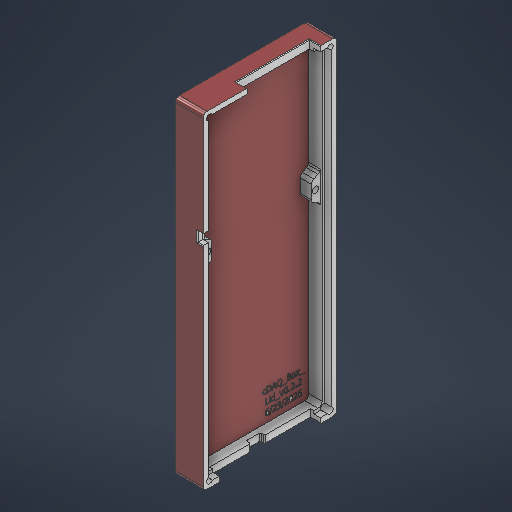
# Autodesk Inventor part: cDAQ_Box_Lid_v0.2.2ipt
Saved by Autodesk Inventor 2027 (Build 310192000, 192)
## iProperties
Created: 2026-05-08
Part Number: cDAQ_Box_Lid_v0.2.2ipt
Material: Generic
Document SubType Name: Modeling
Designer: giese
Density: 1 g/cm^3
Appearance: Default
Author: giese
Autodesk Inventor part; units mm, degrees
(part 1 of 2)
ref_plane "YZ Plane" through (0, 0, 0) normal (1, 0, 0) x (0, 1, 0)
ref_plane "XZ Plane" through (0, 0, 0) normal (0, 1, 0) x (-1, 0, 0)
ref_plane "XY Plane" through (0, 0, 0) normal (0, 0, 1) x (1, 0, 0)
sketch "Sketch1" plane through (0, 0, 0) normal (1, 0, 0) x (0, 1, 0)
  line L0 (50.7569, 48.4212) -> (-204.2591, 48.4212)
  line L1 (-204.2591, 48.4212) -> (-204.2591, -55.7188)
  line L2 (-204.2591, -55.7188) -> (50.7569, -55.7188)
  line L3 (50.7569, -55.7188) -> (50.7569, 48.4212)
  point P0 (0, 0)
  dimension "d0" = 104.14
  dimension "d1" = 255.016
  constraints: 8 end point, 2 parallel, 1 horizontal, 1 perpendicular
  measures "d0" distance of L2.end L0.start
  measures "d1" distance of L0.start L0.end
extrude "Extrusion1" add sketch "Sketch1" along normal blind 21.59
sketch "Sketch2" plane through (21.59, 0, 0) normal (1, 0, 0) x (0, 0, -1)
  line L0 (-42.0712, 44.4069) -> (49.3688, 44.4069)
  line L1 (49.3688, 44.4069) -> (49.3688, -197.9091)
  line L2 (49.3688, -197.9091) -> (-42.0712, -197.9091)
  line L3 (-42.0712, -197.9091) -> (-42.0712, 44.4069)
  line L4 (-48.4212, 50.7569) -> (-48.4212, -204.2591) projected
  line L5 (-48.4212, -204.2591) -> (55.7188, -204.2591) projected
  point P0 (0, 0)
  dimension "d4" = 91.44
  dimension "d5" = 242.316
  dimension "d6" = 6.35
  dimension "d7" = 6.35
  constraints: 8 end point, 2 parallel, 1 horizontal, 1 perpendicular
  measures "d4" distance of L0.start L0.end
  measures "d5" distance of L0.end L1.end
  measures "d6" distance between parallel lines of L4 L3
  measures "d7" distance between parallel lines of L5 L2
extrude "Extrusion2" cut sketch "Sketch2" against normal blind 15.24
sketch "Sketch3" plane through (0, 0, 0) normal (-1, 0, 0) x (0, 0, 1)
  circle A0 centre (-32.8588, 7.3229) radius 2
  line L0 (-55.7188, -204.2591) -> (-55.7188, 50.7569) projected
  line L1 (-55.7188, 50.7569) -> (48.4212, 50.7569) projected
  circle A1 centre (-14.36, 7.3229) radius 2
  circle A2 centre (4.1389, 7.3229) radius 2
  point P0 (0, 0)
  dimension "d10" = 22.86
  dimension "d11" = 43.434
  dimension "d12" = 43.434
  dimension "d13" = 18.4988
  dimension "d14" = 4
  dimension "d15" = 4
  dimension "d16" = 43.434
  dimension "d17" = 18.4988
  dimension "d18" = 36.9976
  dimension "d21" = 4
  constraints: 3 centre point
  measures "d10" distance from line of L0 A0.centre
  measures "d11" distance from line of L1 A0.centre
  measures "d12" distance from line of L1 A1.centre
  measures "d13" distance of A0.centre A1.centre
  measures "d14" diameter of A1
  measures "d15" diameter of A2
  measures "d16" distance from line of L1 A2.centre
  measures "d17" distance of A1.centre A2.centre
  measures "d18" distance of A0.centre A2.centre
  measures "d21" diameter of A0
extrude "Extrusion3" [suppressed]
sketch "Sketch6" plane through (0, 50.7569, 48.4212) normal (0, 1, 0) x (1, 0, 0)
  line L0 (21.59, 6.35) -> (21.59, 97.79) projected
  line L1 (12.954, 34.29) -> (21.59, 34.29)
  line L2 (21.59, 34.29) -> (21.59, 91.44)
  line L3 (21.59, 91.44) -> (12.954, 91.44)
  line L4 (12.954, 91.44) -> (12.954, 34.29)
  line L5 (0, 104.14) -> (21.59, 104.14) projected
  point P0 (0, 48.4212)
  point P1 (17.272, 91.44)
  point P2 (17.272, 34.29)
  dimension "d30" = 8.636
  dimension "d32" = 12.7
  dimension "d220" = 69.85
  constraints: 8 end point, 2 midpoint, 2 parallel, 1 horizontal, 1 perpendicular, 1 point on line
  measures "d30" distance between parallel lines of L0 L4
  measures "d32" distance between parallel lines of L5 L3
  measures "d220" distance between parallel lines of L5 L1
extrude "Extrusion5" cut sketch "Sketch6" against normal blind 6.35
fillet "Fillet1" radius 3.175 4 edges at (10.795, 50.7569, -55.7188) (10.795, 50.7569, 48.4212) (10.795, -204.2591, 48.4212) (10.795, -204.2591, -55.7188)
sketch "Sketch7" plane through (21.59, 0, 0) normal (1, 0, 0) x (0, 0, -1)
  line L0 (-42.0712, -197.9091) -> (-42.0712, 44.4069) projected
  line L1 (-42.0712, 44.4069) -> (-42.3252, 44.4069)
  line L2 (-42.3252, 46.6929) -> (-44.2302, 46.6929)
  line L3 (-44.2302, 46.6929) -> (-44.2302, 51.0109)
  line L4 (-42.0712, -190.1621) -> (-42.0712, -197.9091)
  line L5 (49.3688, -197.9091) -> (-42.0712, -197.9091) projected
  line L6 (-40.4202, -200.1951) -> (-44.2302, -200.1951)
  line L7 (-44.2302, -200.1951) -> (-44.2302, -190.1621)
  line L8 (49.3688, 44.4069) -> (49.3688, -197.9091) projected
  line L9 (49.3688, -192.7021) -> (49.3688, -197.9091)
  line L10 (49.3688, -197.9091) -> (43.9078, -197.9091)
  line L11 (49.3688, -197.9091) -> (49.3688, -192.7021)
  line L12 (51.5278, -192.7021) -> (51.5278, -200.1951)
  line L13 (51.5278, -200.1951) -> (43.9078, -200.1951)
  line L14 (-42.0712, 44.4069) -> (49.3688, 44.4069) projected
  line L15 (42.0028, 44.4069) -> (49.3688, 44.4069)
  line L16 (51.5278, 48.4709) -> (51.5278, 46.6929)
  line L17 (51.5278, 46.6929) -> (42.0028, 46.6929)
  line L18 (-42.3252, 46.6929) -> (42.0028, 46.6929)
  line L19 (42.0028, 44.4069) -> (-42.3252, 44.4069)
  line L20 (51.5278, 48.4709) -> (51.5278, -192.7021)
  line L21 (44.2888, -195.2421) -> (44.2888, 44.4069)
  line L22 (43.9078, -197.9091) -> (-40.4202, -197.9091)
  line L23 (-40.4202, -200.1951) -> (43.9078, -200.1951)
  line L24 (-44.2302, -190.1621) -> (-44.2302, 51.0109)
  line L25 (-42.0712, 44.4069) -> (-42.0712, -190.1621)
  point P0 (0, 0)
  point P1 (-42.0712, 51.0109)
  point P2 (-44.2302, 48.9789)
  point P3 (49.3688, 48.4709)
  point P4 (51.5278, 46.6929)
  point P5 (-44.2302, 46.6929)
  point P6 (-42.0712, 50.7569)
  point P7 (46.8288, 50.7569)
  dimension "d34" = 2.286
  dimension "d35" = 2.159
  dimension "d38" = 2.159
  dimension "d39" = 2.286
  dimension "d42" = 2.286
  dimension "d43" = 2.159
  dimension "d46" = 2.286
  dimension "d47" = 2.159
  constraints: 44 end point, 7 point on line, 4 parallel, 4 perpendicular, 2 collinear, 2 horizontal, 2 vertical, 3 other
  measures "d34" distance between parallel lines of L2 L1
  measures "d35" distance between parallel lines of L0 L3
  measures "d38" distance between parallel lines of L7 L0
  measures "d39" distance between parallel lines of L5 L6
  measures "d42" distance between parallel lines of L5 L13
  measures "d46" distance between parallel lines of L14 L17
extrude "Extrusion6" cut sketch "Sketch7" against normal blind 5 contours L0 L14 L8 L5 | L18 L17 L20 L12 L13 L23 L6 L7 L24 L2
fillet "Fillet2" radius 3.175 6 edges at (11.47, 44.4069, 42.0712) (11.47, 44.4069, -49.3688) (11.47, -197.9091, 42.0712) (19.09, -200.1951, 44.2302) (11.47, -197.9091, -49.3688) (19.09, -200.1951, -51.5278)
sketch "Sketch11" plane through (16.59, 0, 0) normal (1, 0, 0) x (0, 0, -1)
  circle A0 centre (50.6388, 45.6769) radius 2.4005
  line L0 (52.5438, 50.7569) -> (43.0188, 50.7569) projected
  line L1 (55.7188, -201.0841) -> (55.7188, 47.5819) projected
  arc A1 (46.9238, 45.7719) -> (43.7488, 48.9469) centre (43.7488, 45.7719) ccw projected
  circle A2 centre (-43.3412, 45.6769) radius 2.4005
  line L2 (-48.4212, 47.5819) -> (-48.4212, -201.0841) projected
  line L3 (-14.1312, 50.7569) -> (-45.2462, 50.7569) projected
  circle A3 centre (50.6388, -199.1791) radius 2.4005
  line L4 (-45.2462, -204.2591) -> (52.5438, -204.2591) projected
  circle A4 centre (-43.3412, -199.1791) radius 2.4005
  circle A5 centre (45.5588, -50.8431) radius 2.4005
  circle A6 centre (-38.2612, -50.8431) radius 2.4005
  point P0 (0, 0)
  point P1 (45.9939, 48.017)
  point P2 (48.5528, -43.2993)
  point P3 (45.3778, -46.4743)
  point P4 (-30.4007, -42.8803)
  point P5 (-33.5757, -46.0553)
  point P6 (46.8288, 50.7569)
  point P7 (-42.0712, 50.7569)
  dimension "d58" = 4.801
  dimension "d59" = 5.08
  dimension "d60" = 5.08
  dimension "d61" = 4.801
  dimension "d62" = 4.801
  dimension "d63" = 5.08
  dimension "d64" = 5.08
  dimension "d65" = 4.801
  dimension "d66" = 5.08
  dimension "d67" = 5.08
  dimension "d76" = 5.08
  dimension "d77" = 5.08
  dimension "d114" = 4.801
  dimension "d115" = 101.6
  dimension "d116" = 10.16
  dimension "d117" = 4.801
  dimension "d118" = 101.6
  dimension "d119" = 10.16
  constraints: 6 centre point, 1 point on circle
  measures "d58" diameter of A0
  measures "d59" distance from line of L2 A2.centre
  measures "d60" distance from line of L3 A2.centre
  measures "d61" diameter of A2
  measures "d62" diameter of A3
  measures "d63" distance from line of L1 A3.centre
  measures "d64" distance from line of L4 A3.centre
  measures "d65" diameter of A4
  measures "d66" distance from line of L2 A4.centre
  measures "d67" distance from line of L4 A4.centre
  measures "d76" distance from line of L1 A0.centre
  measures "d77" distance from line of L0 A0.centre
  measures "d114" diameter of A5
  measures "d115" distance from line of A5.centre L0
  measures "d116" distance from line of L1 A5.centre
  measures "d117" diameter of A6
  measures "d118" distance from line of A6.centre L3
  measures "d119" distance from line of L2 A6.centre
extrude "Extrusion8" cut sketch "Sketch11" along normal blind 5.08 and the other way blind 17.78
sketch "Sketch13" plane through (6.35, 0, 0) normal (1, 0, 0) x (0, 0, -1)
  line L0 (15.5343, -173.5179) -> (43.4772, -173.5179) construction
  line L1 (43.4772, -173.5179) -> (43.4772, -195.7179) construction
  line L2 (43.4772, -195.7179) -> (15.5343, -195.7179) construction
  line L3 (15.5343, -195.7179) -> (15.5343, -173.5179) construction
  spline S0 degree 2 poles (15.0006, -178.2641) (14.6449, -178.2641) (14.0558, -178.0455) (13.8446, -177.8232) knots 0 0 0 1 2 2 2
  spline S1 degree 2 poles (13.8446, -177.8232) (13.6334, -177.6046) (13.4, -176.9303) (13.4, -176.4783) knots 0 0 0 1 2 2 2
  spline S2 degree 2 poles (13.4, -176.4783) (13.4, -176.0262) (13.6408, -175.3667) (13.8446, -175.1444) knots 0 0 0 1 2 2 2
  spline S3 degree 2 poles (13.8446, -175.1444) (14.0484, -174.9184) (14.6523, -174.6776) (15.0006, -174.6776) knots 0 0 0 1 2 2 2
  spline S4 degree 2 poles (15.0006, -174.6776) (15.2821, -174.6776) (15.8083, -174.8369) (16.012, -174.9407) knots 0 0 0 1 2 2 2
  line L4 (16.012, -174.9407) -> (16.012, -175.5891)
  line L5 (16.012, -175.5891) -> (15.9787, -175.5891)
  spline S5 degree 2 poles (15.9787, -175.5891) (15.9157, -175.5372) (15.723, -175.4038) (15.586, -175.3334) knots 0 0 0 1 2 2 2
  spline S6 degree 2 poles (15.586, -175.3334) (15.4637, -175.2741) (15.1376, -175.1815) (14.9894, -175.1815) knots 0 0 0 1 2 2 2
  spline S7 degree 2 poles (14.9894, -175.1815) (14.5411, -175.1815) (13.9965, -175.8595) (13.9965, -176.4783) knots 0 0 0 1 2 2 2
  spline S8 degree 2 poles (13.9965, -176.4783) (13.9965, -177.0822) (14.5226, -177.7602) (14.9894, -177.7602) knots 0 0 0 1 2 2 2
  spline S9 degree 2 poles (14.9894, -177.7602) (15.271, -177.7602) (15.7823, -177.5268) (15.9787, -177.3452) knots 0 0 0 1 2 2 2
  line L6 (15.9787, -177.3452) -> (16.012, -177.3452)
  line L7 (16.012, -177.3452) -> (16.012, -177.9936)
  spline S10 degree 2 poles (16.012, -177.9936) (15.9268, -178.0344) (15.6675, -178.1492) (15.5637, -178.1752) knots 0 0 0 1 2 2 2
  spline S11 degree 2 poles (15.5637, -178.1752) (15.4155, -178.2196) (15.1821, -178.2641) (15.0006, -178.2641) knots 0 0 0 1 2 2 2
  spline S12 degree 2 poles (20.1876, -175.904) (20.1876, -176.5301) (19.68, -177.5379) (19.2539, -177.8195) knots 0 0 0 1 2 2 2
  spline S13 degree 2 poles (19.2539, -177.8195) (18.9057, -178.0381) (18.1906, -178.1863) (17.6348, -178.1863) knots 0 0 0 1 2 2 2
  line L8 (17.6348, -178.1863) -> (16.5826, -178.1863)
  line L9 (16.5826, -178.1863) -> (16.5826, -173.6143)
  line L10 (16.5826, -173.6143) -> (17.6237, -173.6143)
  spline S14 degree 2 poles (17.6237, -173.6143) (18.2684, -173.6143) (19.002, -173.8069) (19.2613, -173.9774) knots 0 0 0 1 2 2 2
  spline S15 degree 2 poles (19.2613, -173.9774) (19.7022, -174.2701) (20.1876, -175.2371) (20.1876, -175.904) knots 0 0 0 1 2 2 2
  spline S16 degree 2 poles (19.554, -175.8966) (19.554, -175.3705) (19.2058, -174.6257) (18.8612, -174.4146) knots 0 0 0 1 2 2 2
  spline S17 degree 2 poles (18.8612, -174.4146) (18.6167, -174.2701) (18.0646, -174.1404) (17.6534, -174.1404) knots 0 0 0 1 2 2 2
  line L11 (17.6534, -174.1404) -> (17.1902, -174.1404)
  line L12 (17.1902, -174.1404) -> (17.1902, -177.6602)
  line L13 (17.1902, -177.6602) -> (17.6534, -177.6602)
  spline S18 degree 2 poles (17.6534, -177.6602) (18.0572, -177.6602) (18.6685, -177.5305) (18.9168, -177.3563) knots 0 0 0 1 2 2 2
  spline S19 degree 2 poles (18.9168, -177.3563) (19.2354, -177.1415) (19.554, -176.4301) (19.554, -175.8966) knots 0 0 0 1 2 2 2
  line L14 (20.3543, -178.1863) -> (21.8956, -173.6143)
  line L15 (21.8956, -173.6143) -> (22.644, -173.6143)
  line L16 (22.644, -173.6143) -> (24.1853, -178.1863)
  line L17 (24.1853, -178.1863) -> (23.5443, -178.1863)
  line L18 (23.5443, -178.1863) -> (23.1294, -176.908)
  line L19 (23.1294, -176.908) -> (21.3843, -176.908)
  line L20 (21.3843, -176.908) -> (20.9694, -178.1863)
  line L21 (20.9694, -178.1863) -> (20.3543, -178.1863)
  line L22 (22.9627, -176.3893) -> (22.255, -174.2367)
  line L23 (22.255, -174.2367) -> (21.551, -176.3893)
  line L24 (21.551, -176.3893) -> (22.9627, -176.3893)
  spline S20 degree 2 poles (28.4165, -179.3052) (28.2497, -179.3459) (27.8866, -179.3904) (27.7051, -179.3904) knots 0 0 0 1 2 2 2
  spline S21 degree 2 poles (27.7051, -179.3904) (27.1901, -179.3904) (26.5491, -178.8161) (26.5195, -178.2826) knots 0 0 0 1 2 2 2
  spline S22 degree 2 poles (26.5195, -178.2826) (26.4787, -178.2826) (26.4083, -178.2826) (26.3787, -178.2826) knots 0 0 0 1 2 2 2
  spline S23 degree 2 poles (26.3787, -178.2826) (25.9156, -178.2826) (25.1709, -177.9677) (24.9041, -177.6602) knots 0 0 0 1 2 2 2
  spline S24 degree 2 poles (24.9041, -177.6602) (24.641, -177.3563) (24.3595, -176.4671) (24.3595, -175.904) knots 0 0 0 1 2 2 2
  spline S25 degree 2 poles (24.3595, -175.904) (24.3595, -175.326) (24.6447, -174.4516) (24.9078, -174.1404) knots 0 0 0 1 2 2 2
  spline S26 degree 2 poles (24.9078, -174.1404) (25.1746, -173.8329) (25.9193, -173.5179) (26.3787, -173.5179) knots 0 0 0 1 2 2 2
  spline S27 degree 2 poles (26.3787, -173.5179) (26.8455, -173.5179) (27.5939, -173.844) (27.8533, -174.1404) knots 0 0 0 1 2 2 2
  spline S28 degree 2 poles (27.8533, -174.1404) (28.1126, -174.4405) (28.4016, -175.3334) (28.4016, -175.904) knots 0 0 0 1 2 2 2
  spline S29 degree 2 poles (28.4016, -175.904) (28.4016, -176.7932) (27.7088, -177.9492) (27.1049, -178.1529) knots 0 0 0 1 2 2 2
  spline S30 degree 2 poles (27.1049, -178.1529) (27.1197, -178.3234) (27.2086, -178.5975) (27.279, -178.6753) knots 0 0 0 1 2 2 2
  spline S31 degree 2 poles (27.279, -178.6753) (27.3642, -178.7717) (27.5976, -178.8606) (27.8051, -178.8606) knots 0 0 0 1 2 2 2
  spline S32 degree 2 poles (27.8051, -178.8606) (27.9274, -178.8606) (28.2608, -178.7828) (28.3349, -178.7531) knots 0 0 0 1 2 2 2
  line L25 (28.3349, -178.7531) -> (28.4165, -178.7531)
  line L26 (28.4165, -178.7531) -> (28.4165, -179.3052)
  spline S33 degree 2 poles (27.7681, -175.904) (27.7681, -175.4483) (27.5717, -174.748) (27.3939, -174.5183) knots 0 0 0 1 2 2 2
  spline S34 degree 2 poles (27.3939, -174.5183) (27.2123, -174.2812) (26.701, -174.0441) (26.3824, -174.0441) knots 0 0 0 1 2 2 2
  spline S35 degree 2 poles (26.3824, -174.0441) (26.0527, -174.0441) (25.5562, -174.2738) (25.3672, -174.5183) knots 0 0 0 1 2 2 2
  spline S36 degree 2 poles (25.3672, -174.5183) (25.1857, -174.7517) (24.993, -175.4594) (24.993, -175.904) knots 0 0 0 1 2 2 2
  spline S37 degree 2 poles (24.993, -175.904) (24.993, -176.8043) (25.7488, -177.7639) (26.3824, -177.7639) knots 0 0 0 1 2 2 2
  spline S38 degree 2 poles (26.3824, -177.7639) (27.016, -177.7639) (27.7681, -176.8043) (27.7681, -175.904) knots 0 0 0 1 2 2 2
  line L27 (32.0844, -179.1051) -> (28.5572, -179.1051)
  line L28 (28.5572, -179.1051) -> (28.5572, -178.7087)
  line L29 (28.5572, -178.7087) -> (32.0844, -178.7087)
  line L30 (32.0844, -178.7087) -> (32.0844, -179.1051)
  spline S39 degree 2 poles (35.6005, -176.7821) (35.6005, -177.1229) (35.3411, -177.6453) (35.1263, -177.8158) knots 0 0 0 1 2 2 2
  spline S40 degree 2 poles (35.1263, -177.8158) (34.8669, -178.0158) (34.2778, -178.1863) (33.811, -178.1863) knots 0 0 0 1 2 2 2
  line L31 (33.811, -178.1863) -> (32.4994, -178.1863)
  line L32 (32.4994, -178.1863) -> (32.4994, -173.6143)
  line L33 (32.4994, -173.6143) -> (33.7109, -173.6143)
  spline S41 degree 2 poles (33.7109, -173.6143) (34.2, -173.6143) (34.6891, -173.6773) (34.9114, -173.7995) knots 0 0 0 1 2 2 2
  spline S42 degree 2 poles (34.9114, -173.7995) (35.1596, -173.9292) (35.3856, -174.3553) (35.3856, -174.6443) knots 0 0 0 1 2 2 2
  spline S43 degree 2 poles (35.3856, -174.6443) (35.3856, -174.9666) (35.0447, -175.4779) (34.7446, -175.6224) knots 0 0 0 1 2 2 2
  line L34 (34.7446, -175.6224) -> (34.7446, -175.6446)
  spline S44 degree 2 poles (34.7446, -175.6446) (35.1522, -175.7558) (35.6005, -176.3449) (35.6005, -176.7821) knots 0 0 0 1 2 2 2
  spline S45 degree 2 poles (34.9669, -176.808) (34.9669, -176.5487) (34.8187, -176.2152) (34.5964, -176.0966) knots 0 0 0 1 2 2 2
  spline S46 degree 2 poles (34.5964, -176.0966) (34.4519, -176.0225) (34.1111, -175.9781) (33.7962, -175.9781) knots 0 0 0 1 2 2 2
  line L35 (33.7962, -175.9781) -> (33.107, -175.9781)
  line L36 (33.107, -175.9781) -> (33.107, -177.6676)
  line L37 (33.107, -177.6676) -> (33.5998, -177.6676)
  spline S47 degree 2 poles (33.5998, -177.6676) (33.9999, -177.6676) (34.4594, -177.5935) (34.6372, -177.4749) knots 0 0 0 1 2 2 2
  spline S48 degree 2 poles (34.6372, -177.4749) (34.8076, -177.3526) (34.9669, -177.0488) (34.9669, -176.808) knots 0 0 0 1 2 2 2
  spline S49 degree 2 poles (34.752, -174.7295) (34.752, -174.5665) (34.6409, -174.3219) (34.5186, -174.2515) knots 0 0 0 1 2 2 2
  spline S50 degree 2 poles (34.5186, -174.2515) (34.3704, -174.17) (34.011, -174.133) (33.6887, -174.133) knots 0 0 0 1 2 2 2
  line L38 (33.6887, -174.133) -> (33.107, -174.133)
  line L39 (33.107, -174.133) -> (33.107, -175.4705)
  line L40 (33.107, -175.4705) -> (33.7962, -175.4705)
  spline S51 degree 2 poles (33.7962, -175.4705) (34.0814, -175.4705) (34.3519, -175.4112) (34.4964, -175.3186) knots 0 0 0 1 2 2 2
  spline S52 degree 2 poles (34.4964, -175.3186) (34.6372, -175.2297) (34.752, -174.9444) (34.752, -174.7295) knots 0 0 0 1 2 2 2
  spline S53 degree 2 poles (38.9795, -176.4708) (38.9795, -177.3378) (38.1459, -178.2826) (37.4493, -178.2826) knots 0 0 0 1 2 2 2
  spline S54 degree 2 poles (37.4493, -178.2826) (36.7342, -178.2826) (35.9154, -177.3082) (35.9154, -176.4708) knots 0 0 0 1 2 2 2
  spline S55 degree 2 poles (35.9154, -176.4708) (35.9154, -175.6113) (36.7602, -174.6591) (37.4493, -174.6591) knots 0 0 0 1 2 2 2
  spline S56 degree 2 poles (37.4493, -174.6591) (38.1459, -174.6591) (38.9795, -175.6076) (38.9795, -176.4708) knots 0 0 0 1 2 2 2
  spline S57 degree 2 poles (38.383, -176.4708) (38.383, -175.8039) (37.8976, -175.1556) (37.4493, -175.1556) knots 0 0 0 1 2 2 2
  spline S58 degree 2 poles (37.4493, -175.1556) (37.001, -175.1556) (36.5119, -175.8039) (36.5119, -176.4708) knots 0 0 0 1 2 2 2
  spline S59 degree 2 poles (36.5119, -176.4708) (36.5119, -177.1192) (37.001, -177.7861) (37.4493, -177.7861) knots 0 0 0 1 2 2 2
  spline S60 degree 2 poles (37.4493, -177.7861) (37.8939, -177.7861) (38.383, -177.1303) (38.383, -176.4708) knots 0 0 0 1 2 2 2
  line L41 (42.2362, -178.1863) -> (41.5285, -178.1863)
  line L42 (41.5285, -178.1863) -> (40.6949, -176.8969)
  line L43 (40.6949, -176.8969) -> (39.839, -178.1863)
  line L44 (39.839, -178.1863) -> (39.1833, -178.1863)
  line L45 (39.1833, -178.1863) -> (40.3726, -176.4857)
  line L46 (40.3726, -176.4857) -> (39.1944, -174.7554)
  line L47 (39.1944, -174.7554) -> (39.902, -174.7554)
  line L48 (39.902, -174.7554) -> (40.732, -176.0337)
  line L49 (40.732, -176.0337) -> (41.5804, -174.7554)
  line L50 (41.5804, -174.7554) -> (42.2362, -174.7554)
  line L51 (42.2362, -174.7554) -> (41.0543, -176.4486)
  line L52 (41.0543, -176.4486) -> (42.2362, -178.1863)
  line L53 (45.7449, -179.1051) -> (42.2177, -179.1051)
  line L54 (42.2177, -179.1051) -> (42.2177, -178.7087)
  line L55 (42.2177, -178.7087) -> (45.7449, -178.7087)
  line L56 (45.7449, -178.7087) -> (45.7449, -179.1051)
  line L57 (18.2665, -185.714) -> (15.6175, -185.714)
  line L58 (15.6175, -185.714) -> (15.6175, -181.142)
  line L59 (15.6175, -181.142) -> (16.2251, -181.142)
  line L60 (16.2251, -181.142) -> (16.2251, -185.173)
  line L61 (16.2251, -185.173) -> (18.2665, -185.173)
  line L62 (18.2665, -185.173) -> (18.2665, -185.714)
  line L63 (19.2891, -185.714) -> (18.7111, -185.714)
  line L64 (18.7111, -185.714) -> (18.7111, -182.2831)
  line L65 (18.7111, -182.2831) -> (19.2891, -182.2831)
  line L66 (19.2891, -182.2831) -> (19.2891, -185.714)
  line L67 (19.3299, -181.7125) -> (18.6741, -181.7125)
  line L68 (18.6741, -181.7125) -> (18.6741, -181.1123)
  line L69 (18.6741, -181.1123) -> (19.3299, -181.1123)
  line L70 (19.3299, -181.1123) -> (19.3299, -181.7125)
  line L71 (22.7756, -185.714) -> (22.1976, -185.714)
  line L72 (22.1976, -185.714) -> (22.1976, -185.3657)
  spline S61 degree 2 poles (22.1976, -185.3657) (22.0642, -185.4768) (21.8678, -185.625) (21.7344, -185.688) knots 0 0 0 1 2 2 2
  spline S62 degree 2 poles (21.7344, -185.688) (21.6122, -185.7473) (21.3491, -185.8103) (21.175, -185.8103) knots 0 0 0 1 2 2 2
  spline S63 degree 2 poles (21.175, -185.8103) (20.8934, -185.8103) (20.4192, -185.5769) (20.2524, -185.3509) knots 0 0 0 1 2 2 2
  spline S64 degree 2 poles (20.2524, -185.3509) (20.0857, -185.1249) (19.9005, -184.4579) (19.9005, -184.0245) knots 0 0 0 1 2 2 2
  spline S65 degree 2 poles (19.9005, -184.0245) (19.9005, -183.5724) (20.1339, -182.913) (20.3377, -182.6647) knots 0 0 0 1 2 2 2
  spline S66 degree 2 poles (20.3377, -182.6647) (20.5266, -182.4424) (21.0564, -182.1868) (21.3491, -182.1868) knots 0 0 0 1 2 2 2
  spline S67 degree 2 poles (21.3491, -182.1868) (21.6048, -182.1868) (21.9864, -182.3016) (22.1976, -182.4202) knots 0 0 0 1 2 2 2
  line L73 (22.1976, -182.4202) -> (22.1976, -180.9382)
  line L74 (22.1976, -180.9382) -> (22.7756, -180.9382)
  line L75 (22.7756, -180.9382) -> (22.7756, -185.714)
  line L76 (22.1976, -184.8803) -> (22.1976, -182.8981)
  spline S68 degree 2 poles (22.1976, -182.8981) (21.9827, -182.7944) (21.6418, -182.7166) (21.4455, -182.7166) knots 0 0 0 1 2 2 2
  spline S69 degree 2 poles (21.4455, -182.7166) (21.0009, -182.7166) (20.497, -183.3835) (20.497, -184.0133) knots 0 0 0 1 2 2 2
  spline S70 degree 2 poles (20.497, -184.0133) (20.497, -184.621) (20.8823, -185.2619) (21.3084, -185.2619) knots 0 0 0 1 2 2 2
  spline S71 degree 2 poles (21.3084, -185.2619) (21.5344, -185.2619) (21.9938, -185.0545) (22.1976, -184.8803) knots 0 0 0 1 2 2 2
  line L77 (26.6732, -186.6328) -> (23.1461, -186.6328)
  line L78 (23.1461, -186.6328) -> (23.1461, -186.2364)
  line L79 (23.1461, -186.2364) -> (26.6732, -186.2364)
  line L80 (26.6732, -186.2364) -> (26.6732, -186.6328)
  line L81 (29.7373, -182.2831) -> (28.4442, -185.714)
  line L82 (28.4442, -185.714) -> (27.9255, -185.714)
  line L83 (27.9255, -185.714) -> (26.6436, -182.2831)
  line L84 (26.6436, -182.2831) -> (27.2698, -182.2831)
  line L85 (27.2698, -182.2831) -> (28.2071, -184.9248)
  line L86 (28.2071, -184.9248) -> (29.1371, -182.2831)
  line L87 (29.1371, -182.2831) -> (29.7373, -182.2831)
  spline S72 degree 2 poles (32.9347, -183.428) (32.9347, -184.658) (32.2197, -185.8103) (31.475, -185.8103) knots 0 0 0 1 2 2 2
  spline S73 degree 2 poles (31.475, -185.8103) (30.7191, -185.8103) (30.0115, -184.6358) (30.0115, -183.4317) knots 0 0 0 1 2 2 2
  spline S74 degree 2 poles (30.0115, -183.4317) (30.0115, -182.1942) (30.7265, -181.0493) (31.475, -181.0493) knots 0 0 0 1 2 2 2
  spline S75 degree 2 poles (31.475, -181.0493) (32.2271, -181.0493) (32.9347, -182.2349) (32.9347, -183.428) knots 0 0 0 1 2 2 2
  spline S76 degree 2 poles (32.1493, -184.821) (32.2382, -184.595) (32.3123, -183.8985) (32.3123, -183.428) knots 0 0 0 1 2 2 2
  spline S77 degree 2 poles (32.3123, -183.428) (32.3123, -182.9574) (32.2382, -182.2646) (32.1456, -182.0312) knots 0 0 0 1 2 2 2
  spline S78 degree 2 poles (32.1456, -182.0312) (32.0529, -181.7977) (31.7306, -181.5569) (31.475, -181.5569) knots 0 0 0 1 2 2 2
  spline S79 degree 2 poles (31.475, -181.5569) (31.2193, -181.5569) (30.8896, -181.7977) (30.7932, -182.0386) knots 0 0 0 1 2 2 2
  spline S80 degree 2 poles (30.7932, -182.0386) (30.7006, -182.272) (30.6339, -182.9833) (30.6339, -183.4317) knots 0 0 0 1 2 2 2
  spline S81 degree 2 poles (30.6339, -183.4317) (30.6339, -183.9133) (30.6932, -184.558) (30.7895, -184.8099) knots 0 0 0 1 2 2 2
  spline S82 degree 2 poles (30.7895, -184.8099) (30.8784, -185.047) (31.2082, -185.3027) (31.475, -185.3027) knots 0 0 0 1 2 2 2
  spline S83 degree 2 poles (31.475, -185.3027) (31.7269, -185.3027) (32.0566, -185.0619) (32.1493, -184.821) knots 0 0 0 1 2 2 2
  line L88 (34.502, -185.714) -> (33.7684, -185.714)
  line L89 (33.7684, -185.714) -> (33.7684, -184.8396)
  line L90 (33.7684, -184.8396) -> (34.502, -184.8396)
  line L91 (34.502, -184.8396) -> (34.502, -185.714)
  line L92 (38.244, -185.714) -> (35.4245, -185.714)
  line L93 (35.4245, -185.714) -> (35.4245, -185.0656)
  spline S84 degree 2 poles (35.4245, -185.0656) (35.7283, -184.7803) (36.2693, -184.2505) (36.5286, -183.9652) knots 0 0 0 1 2 2 2
  spline S85 degree 2 poles (36.5286, -183.9652) (37.051, -183.3909) (37.4326, -182.7018) (37.4326, -182.335) knots 0 0 0 1 2 2 2
  spline S86 degree 2 poles (37.4326, -182.335) (37.4326, -182.1423) (37.3141, -181.8533) (37.2066, -181.7607) knots 0 0 0 1 2 2 2
  spline S87 degree 2 poles (37.2066, -181.7607) (37.0992, -181.6681) (36.8176, -181.5754) (36.6472, -181.5754) knots 0 0 0 1 2 2 2
  spline S88 degree 2 poles (36.6472, -181.5754) (36.4841, -181.5754) (36.1507, -181.6569) (35.9988, -181.7199) knots 0 0 0 1 2 2 2
  spline S89 degree 2 poles (35.9988, -181.7199) (35.8691, -181.7718) (35.6283, -181.92) (35.5542, -181.9719) knots 0 0 0 1 2 2 2
  line L94 (35.5542, -181.9719) -> (35.5208, -181.9719)
  line L95 (35.5208, -181.9719) -> (35.5208, -181.3198)
  spline S90 degree 2 poles (35.5208, -181.3198) (35.7098, -181.2272) (36.3878, -181.0456) (36.6916, -181.0456) knots 0 0 0 1 2 2 2
  spline S91 degree 2 poles (36.6916, -181.0456) (37.3326, -181.0456) (38.0551, -181.7236) (38.0551, -182.3016) knots 0 0 0 1 2 2 2
  spline S92 degree 2 poles (38.0551, -182.3016) (38.0551, -182.5721) (37.9291, -183.0241) (37.818, -183.2168) knots 0 0 0 1 2 2 2
  spline S93 degree 2 poles (37.818, -183.2168) (37.7068, -183.4168) (37.3845, -183.8096) (37.2066, -183.9985) knots 0 0 0 1 2 2 2
  spline S94 degree 2 poles (37.2066, -183.9985) (36.9176, -184.3135) (36.21, -184.9878) (35.9988, -185.1841) knots 0 0 0 1 2 2 2
  line L96 (35.9988, -185.1841) -> (38.244, -185.1841)
  line L97 (38.244, -185.1841) -> (38.244, -185.714)
  line L98 (39.8372, -185.714) -> (39.1036, -185.714)
  line L99 (39.1036, -185.714) -> (39.1036, -184.8396)
  line L100 (39.1036, -184.8396) -> (39.8372, -184.8396)
  line L101 (39.8372, -184.8396) -> (39.8372, -185.714)
  line L102 (43.5793, -185.714) -> (40.7597, -185.714)
  line L103 (40.7597, -185.714) -> (40.7597, -185.0656)
  spline S95 degree 2 poles (40.7597, -185.0656) (41.0636, -184.7803) (41.6045, -184.2505) (41.8638, -183.9652) knots 0 0 0 1 2 2 2
  spline S96 degree 2 poles (41.8638, -183.9652) (42.3863, -183.3909) (42.7679, -182.7018) (42.7679, -182.335) knots 0 0 0 1 2 2 2
  spline S97 degree 2 poles (42.7679, -182.335) (42.7679, -182.1423) (42.6493, -181.8533) (42.5419, -181.7607) knots 0 0 0 1 2 2 2
  spline S98 degree 2 poles (42.5419, -181.7607) (42.4344, -181.6681) (42.1528, -181.5754) (41.9824, -181.5754) knots 0 0 0 1 2 2 2
  spline S99 degree 2 poles (41.9824, -181.5754) (41.8194, -181.5754) (41.4859, -181.6569) (41.334, -181.7199) knots 0 0 0 1 2 2 2
  spline S100 degree 2 poles (41.334, -181.7199) (41.2043, -181.7718) (40.9635, -181.92) (40.8894, -181.9719) knots 0 0 0 1 2 2 2
  line L104 (40.8894, -181.9719) -> (40.8561, -181.9719)
  line L105 (40.8561, -181.9719) -> (40.8561, -181.3198)
  spline S101 degree 2 poles (40.8561, -181.3198) (41.045, -181.2272) (41.7231, -181.0456) (42.0269, -181.0456) knots 0 0 0 1 2 2 2
  spline S102 degree 2 poles (42.0269, -181.0456) (42.6678, -181.0456) (43.3903, -181.7236) (43.3903, -182.3016) knots 0 0 0 1 2 2 2
  spline S103 degree 2 poles (43.3903, -182.3016) (43.3903, -182.5721) (43.2643, -183.0241) (43.1532, -183.2168) knots 0 0 0 1 2 2 2
  spline S104 degree 2 poles (43.1532, -183.2168) (43.042, -183.4168) (42.7197, -183.8096) (42.5419, -183.9985) knots 0 0 0 1 2 2 2
  spline S105 degree 2 poles (42.5419, -183.9985) (42.2529, -184.3135) (41.5452, -184.9878) (41.334, -185.1841) knots 0 0 0 1 2 2 2
  line L106 (41.334, -185.1841) -> (43.5793, -185.1841)
  line L107 (43.5793, -185.1841) -> (43.5793, -185.714)
  spline S106 degree 2 poles (18.3166, -191.7596) (18.3166, -192.1116) (18.0831, -192.7081) (17.8868, -192.9082) knots 0 0 0 1 2 2 2
  spline S107 degree 2 poles (17.8868, -192.9082) (17.683, -193.1194) (17.1717, -193.338) (16.8642, -193.338) knots 0 0 0 1 2 2 2
  spline S108 degree 2 poles (16.8642, -193.338) (16.5567, -193.338) (16.0491, -193.1305) (15.8564, -192.923) knots 0 0 0 1 2 2 2
  spline S109 degree 2 poles (15.8564, -192.923) (15.6193, -192.6748) (15.3525, -191.8411) (15.3525, -191.2335) knots 0 0 0 1 2 2 2
  spline S110 degree 2 poles (15.3525, -191.2335) (15.3525, -190.637) (15.5971, -189.6774) (15.8527, -189.3217) knots 0 0 0 1 2 2 2
  spline S111 degree 2 poles (15.8527, -189.3217) (16.101, -188.9734) (16.8864, -188.5844) (17.4014, -188.5844) knots 0 0 0 1 2 2 2
  spline S112 degree 2 poles (17.4014, -188.5844) (17.5533, -188.5844) (17.8201, -188.6141) (17.9201, -188.6474) knots 0 0 0 1 2 2 2
  line L108 (17.9201, -188.6474) -> (17.9201, -189.2365)
  line L109 (17.9201, -189.2365) -> (17.8942, -189.2365)
  spline S113 degree 2 poles (17.8942, -189.2365) (17.809, -189.192) (17.4978, -189.1142) (17.3199, -189.1142) knots 0 0 0 1 2 2 2
  spline S114 degree 2 poles (17.3199, -189.1142) (16.7493, -189.1142) (16.0491, -189.8849) (15.9824, -190.6407) knots 0 0 0 1 2 2 2
  spline S115 degree 2 poles (15.9824, -190.6407) (16.201, -190.4888) (16.6604, -190.3221) (16.9346, -190.3221) knots 0 0 0 1 2 2 2
  spline S116 degree 2 poles (16.9346, -190.3221) (17.2013, -190.3221) (17.6015, -190.4295) (17.8201, -190.5925) knots 0 0 0 1 2 2 2
  spline S117 degree 2 poles (17.8201, -190.5925) (18.072, -190.7815) (18.3166, -191.3669) (18.3166, -191.7596) knots 0 0 0 1 2 2 2
  spline S118 degree 2 poles (17.6941, -191.7856) (17.6941, -191.504) (17.5459, -191.1224) (17.3829, -190.989) knots 0 0 0 1 2 2 2
  spline S119 degree 2 poles (17.3829, -190.989) (17.2606, -190.8926) (16.9568, -190.8297) (16.7975, -190.8297) knots 0 0 0 1 2 2 2
  spline S120 degree 2 poles (16.7975, -190.8297) (16.5826, -190.8297) (16.1788, -190.9593) (15.9824, -191.0816) knots 0 0 0 1 2 2 2
  spline S121 degree 2 poles (15.9824, -191.0816) (15.9787, -191.1483) (15.9713, -191.2743) (15.9713, -191.3706) knots 0 0 0 1 2 2 2
  spline S122 degree 2 poles (15.9713, -191.3706) (15.9713, -191.8448) (16.1565, -192.4265) (16.2973, -192.5784) knots 0 0 0 1 2 2 2
  spline S123 degree 2 poles (16.2973, -192.5784) (16.427, -192.7229) (16.7086, -192.8378) (16.8679, -192.8378) knots 0 0 0 1 2 2 2
  spline S124 degree 2 poles (16.8679, -192.8378) (17.2384, -192.8378) (17.6941, -192.3117) (17.6941, -191.7856) knots 0 0 0 1 2 2 2
  line L110 (20.7582, -188.4659) -> (18.9686, -194.2346)
  line L111 (18.9686, -194.2346) -> (18.4499, -194.2346)
  line L112 (18.4499, -194.2346) -> (20.2321, -188.4659)
  line L113 (20.2321, -188.4659) -> (20.7582, -188.4659)
  line L114 (24.0816, -193.2416) -> (21.2621, -193.2416)
  line L115 (21.2621, -193.2416) -> (21.2621, -192.5932)
  spline S125 degree 2 poles (21.2621, -192.5932) (21.5659, -192.308) (22.1068, -191.7781) (22.3662, -191.4929) knots 0 0 0 1 2 2 2
  spline S126 degree 2 poles (22.3662, -191.4929) (22.8886, -190.9186) (23.2702, -190.2294) (23.2702, -189.8626) knots 0 0 0 1 2 2 2
  spline S127 degree 2 poles (23.2702, -189.8626) (23.2702, -189.67) (23.1516, -189.381) (23.0442, -189.2884) knots 0 0 0 1 2 2 2
  spline S128 degree 2 poles (23.0442, -189.2884) (22.9367, -189.1957) (22.6551, -189.1031) (22.4847, -189.1031) knots 0 0 0 1 2 2 2
  spline S129 degree 2 poles (22.4847, -189.1031) (22.3217, -189.1031) (21.9882, -189.1846) (21.8363, -189.2476) knots 0 0 0 1 2 2 2
  spline S130 degree 2 poles (21.8363, -189.2476) (21.7067, -189.2995) (21.4658, -189.4477) (21.3917, -189.4996) knots 0 0 0 1 2 2 2
  line L116 (21.3917, -189.4996) -> (21.3584, -189.4996)
  line L117 (21.3584, -189.4996) -> (21.3584, -188.8475)
  spline S131 degree 2 poles (21.3584, -188.8475) (21.5473, -188.7548) (22.2254, -188.5733) (22.5292, -188.5733) knots 0 0 0 1 2 2 2
  spline S132 degree 2 poles (22.5292, -188.5733) (23.1701, -188.5733) (23.8926, -189.2513) (23.8926, -189.8293) knots 0 0 0 1 2 2 2
  spline S133 degree 2 poles (23.8926, -189.8293) (23.8926, -190.0998) (23.7667, -190.5518) (23.6555, -190.7444) knots 0 0 0 1 2 2 2
  spline S134 degree 2 poles (23.6555, -190.7444) (23.5443, -190.9445) (23.222, -191.3372) (23.0442, -191.5262) knots 0 0 0 1 2 2 2
  spline S135 degree 2 poles (23.0442, -191.5262) (22.7552, -191.8411) (22.0475, -192.5154) (21.8363, -192.7118) knots 0 0 0 1 2 2 2
  line L118 (21.8363, -192.7118) -> (24.0816, -192.7118)
  line L119 (24.0816, -192.7118) -> (24.0816, -193.2416)
  spline S136 degree 2 poles (25.9267, -189.1031) (25.76, -189.1031) (25.4302, -189.1846) (25.2709, -189.2476) knots 0 0 0 1 2 2 2
  spline S137 degree 2 poles (25.2709, -189.2476) (25.1227, -189.3106) (24.9041, -189.444) (24.8189, -189.5033) knots 0 0 0 1 2 2 2
  line L120 (24.8189, -189.5033) -> (24.7818, -189.5033)
  line L121 (24.7818, -189.5033) -> (24.7818, -188.8549)
  spline S138 degree 2 poles (24.7818, -188.8549) (24.9819, -188.7474) (25.6673, -188.5733) (25.9748, -188.5733) knots 0 0 0 1 2 2 2
  spline S139 degree 2 poles (25.9748, -188.5733) (26.2861, -188.5733) (26.7492, -188.6993) (26.9382, -188.8326) knots 0 0 0 1 2 2 2
  spline S140 degree 2 poles (26.9382, -188.8326) (27.1382, -188.9771) (27.3457, -189.3958) (27.3457, -189.6774) knots 0 0 0 1 2 2 2
  spline S141 degree 2 poles (27.3457, -189.6774) (27.3457, -190.0553) (26.8492, -190.6259) (26.501, -190.7) knots 0 0 0 1 2 2 2
  line L122 (26.501, -190.7) -> (26.501, -190.7444)
  spline S142 degree 2 poles (26.501, -190.7444) (26.6455, -190.7741) (26.9752, -190.9075) (27.116, -191.0408) knots 0 0 0 1 2 2 2
  spline S143 degree 2 poles (27.116, -191.0408) (27.2568, -191.1705) (27.4346, -191.5855) (27.4346, -191.8856) knots 0 0 0 1 2 2 2
  spline S144 degree 2 poles (27.4346, -191.8856) (27.4346, -192.1931) (27.2234, -192.7155) (27.0308, -192.9156) knots 0 0 0 1 2 2 2
  spline S145 degree 2 poles (27.0308, -192.9156) (26.8307, -193.1231) (26.2638, -193.338) (25.9045, -193.338) knots 0 0 0 1 2 2 2
  spline S146 degree 2 poles (25.9045, -193.338) (25.5599, -193.338) (24.8856, -193.1712) (24.6559, -193.0564) knots 0 0 0 1 2 2 2
  line L123 (24.6559, -193.0564) -> (24.6559, -192.408)
  line L124 (24.6559, -192.408) -> (24.7003, -192.408)
  spline S147 degree 2 poles (24.7003, -192.408) (24.893, -192.5488) (25.5451, -192.8081) (25.8674, -192.8081) knots 0 0 0 1 2 2 2
  spline S148 degree 2 poles (25.8674, -192.8081) (26.0564, -192.8081) (26.4343, -192.6896) (26.5602, -192.5525) knots 0 0 0 1 2 2 2
  spline S149 degree 2 poles (26.5602, -192.5525) (26.6825, -192.4154) (26.8122, -192.0894) (26.8122, -191.8411) knots 0 0 0 1 2 2 2
  spline S150 degree 2 poles (26.8122, -191.8411) (26.8122, -191.5929) (26.6677, -191.2706) (26.538, -191.1779) knots 0 0 0 1 2 2 2
  spline S151 degree 2 poles (26.538, -191.1779) (26.4083, -191.0853) (26.0564, -191.0149) (25.8489, -191.0149) knots 0 0 0 1 2 2 2
  line L125 (25.8489, -191.0149) -> (25.5895, -191.0149)
  line L126 (25.5895, -191.0149) -> (25.5895, -190.5073)
  line L127 (25.5895, -190.5073) -> (25.7933, -190.5073)
  spline S152 degree 2 poles (25.7933, -190.5073) (26.2046, -190.5073) (26.7233, -190.1146) (26.7233, -189.7404) knots 0 0 0 1 2 2 2
  spline S153 degree 2 poles (26.7233, -189.7404) (26.7233, -189.5662) (26.5899, -189.318) (26.4824, -189.2439) knots 0 0 0 1 2 2 2
  spline S154 degree 2 poles (26.4824, -189.2439) (26.3676, -189.1661) (26.086, -189.1031) (25.9267, -189.1031) knots 0 0 0 1 2 2 2
  line L128 (30.0244, -188.4659) -> (28.2349, -194.2346)
  line L129 (28.2349, -194.2346) -> (27.7162, -194.2346)
  line L130 (27.7162, -194.2346) -> (29.4983, -188.4659)
  line L131 (29.4983, -188.4659) -> (30.0244, -188.4659)
  line L132 (33.3478, -193.2416) -> (30.5283, -193.2416)
  line L133 (30.5283, -193.2416) -> (30.5283, -192.5932)
  spline S155 degree 2 poles (30.5283, -192.5932) (30.8321, -192.308) (31.3731, -191.7781) (31.6324, -191.4929) knots 0 0 0 1 2 2 2
  spline S156 degree 2 poles (31.6324, -191.4929) (32.1548, -190.9186) (32.5364, -190.2294) (32.5364, -189.8626) knots 0 0 0 1 2 2 2
  spline S157 degree 2 poles (32.5364, -189.8626) (32.5364, -189.67) (32.4179, -189.381) (32.3104, -189.2884) knots 0 0 0 1 2 2 2
  spline S158 degree 2 poles (32.3104, -189.2884) (32.203, -189.1957) (31.9214, -189.1031) (31.751, -189.1031) knots 0 0 0 1 2 2 2
  spline S159 degree 2 poles (31.751, -189.1031) (31.588, -189.1031) (31.2545, -189.1846) (31.1026, -189.2476) knots 0 0 0 1 2 2 2
  spline S160 degree 2 poles (31.1026, -189.2476) (30.9729, -189.2995) (30.7321, -189.4477) (30.658, -189.4996) knots 0 0 0 1 2 2 2
  line L134 (30.658, -189.4996) -> (30.6247, -189.4996)
  line L135 (30.6247, -189.4996) -> (30.6247, -188.8475)
  spline S161 degree 2 poles (30.6247, -188.8475) (30.8136, -188.7548) (31.4916, -188.5733) (31.7954, -188.5733) knots 0 0 0 1 2 2 2
  spline S162 degree 2 poles (31.7954, -188.5733) (32.4364, -188.5733) (33.1589, -189.2513) (33.1589, -189.8293) knots 0 0 0 1 2 2 2
  spline S163 degree 2 poles (33.1589, -189.8293) (33.1589, -190.0998) (33.0329, -190.5518) (32.9218, -190.7444) knots 0 0 0 1 2 2 2
  spline S164 degree 2 poles (32.9218, -190.7444) (32.8106, -190.9445) (32.4883, -191.3372) (32.3104, -191.5262) knots 0 0 0 1 2 2 2
  spline S165 degree 2 poles (32.3104, -191.5262) (32.0214, -191.8411) (31.3138, -192.5154) (31.1026, -192.7118) knots 0 0 0 1 2 2 2
  line L136 (31.1026, -192.7118) -> (33.3478, -192.7118)
  line L137 (33.3478, -192.7118) -> (33.3478, -193.2416)
  spline S166 degree 2 poles (36.8046, -190.9556) (36.8046, -192.1857) (36.0896, -193.338) (35.3449, -193.338) knots 0 0 0 1 2 2 2
  spline S167 degree 2 poles (35.3449, -193.338) (34.589, -193.338) (33.8814, -192.1635) (33.8814, -190.9593) knots 0 0 0 1 2 2 2
  spline S168 degree 2 poles (33.8814, -190.9593) (33.8814, -189.7219) (34.5964, -188.577) (35.3449, -188.577) knots 0 0 0 1 2 2 2
  spline S169 degree 2 poles (35.3449, -188.577) (36.097, -188.577) (36.8046, -189.7626) (36.8046, -190.9556) knots 0 0 0 1 2 2 2
  spline S170 degree 2 poles (36.0192, -192.3487) (36.1081, -192.1227) (36.1822, -191.4262) (36.1822, -190.9556) knots 0 0 0 1 2 2 2
  spline S171 degree 2 poles (36.1822, -190.9556) (36.1822, -190.4851) (36.1081, -189.7923) (36.0155, -189.5588) knots 0 0 0 1 2 2 2
  spline S172 degree 2 poles (36.0155, -189.5588) (35.9228, -189.3254) (35.6005, -189.0846) (35.3449, -189.0846) knots 0 0 0 1 2 2 2
  spline S173 degree 2 poles (35.3449, -189.0846) (35.0892, -189.0846) (34.7595, -189.3254) (34.6631, -189.5662) knots 0 0 0 1 2 2 2
  spline S174 degree 2 poles (34.6631, -189.5662) (34.5705, -189.7997) (34.5038, -190.511) (34.5038, -190.9593) knots 0 0 0 1 2 2 2
  spline S175 degree 2 poles (34.5038, -190.9593) (34.5038, -191.441) (34.5631, -192.0857) (34.6594, -192.3376) knots 0 0 0 1 2 2 2
  spline S176 degree 2 poles (34.6594, -192.3376) (34.7483, -192.5747) (35.0781, -192.8304) (35.3449, -192.8304) knots 0 0 0 1 2 2 2
  spline S177 degree 2 poles (35.3449, -192.8304) (35.5968, -192.8304) (35.9265, -192.5895) (36.0192, -192.3487) knots 0 0 0 1 2 2 2
  line L138 (40.2095, -193.2416) -> (37.39, -193.2416)
  line L139 (37.39, -193.2416) -> (37.39, -192.5932)
  spline S178 degree 2 poles (37.39, -192.5932) (37.6938, -192.308) (38.2348, -191.7781) (38.4941, -191.4929) knots 0 0 0 1 2 2 2
  spline S179 degree 2 poles (38.4941, -191.4929) (39.0165, -190.9186) (39.3981, -190.2294) (39.3981, -189.8626) knots 0 0 0 1 2 2 2
  spline S180 degree 2 poles (39.3981, -189.8626) (39.3981, -189.67) (39.2796, -189.381) (39.1721, -189.2884) knots 0 0 0 1 2 2 2
  spline S181 degree 2 poles (39.1721, -189.2884) (39.0647, -189.1957) (38.7831, -189.1031) (38.6127, -189.1031) knots 0 0 0 1 2 2 2
  spline S182 degree 2 poles (38.6127, -189.1031) (38.4497, -189.1031) (38.1162, -189.1846) (37.9643, -189.2476) knots 0 0 0 1 2 2 2
  spline S183 degree 2 poles (37.9643, -189.2476) (37.8346, -189.2995) (37.5938, -189.4477) (37.5197, -189.4996) knots 0 0 0 1 2 2 2
  line L140 (37.5197, -189.4996) -> (37.4864, -189.4996)
  line L141 (37.4864, -189.4996) -> (37.4864, -188.8475)
  spline S184 degree 2 poles (37.4864, -188.8475) (37.6753, -188.7548) (38.3533, -188.5733) (38.6571, -188.5733) knots 0 0 0 1 2 2 2
  spline S185 degree 2 poles (38.6571, -188.5733) (39.2981, -188.5733) (40.0206, -189.2513) (40.0206, -189.8293) knots 0 0 0 1 2 2 2
  spline S186 degree 2 poles (40.0206, -189.8293) (40.0206, -190.0998) (39.8946, -190.5518) (39.7835, -190.7444) knots 0 0 0 1 2 2 2
  spline S187 degree 2 poles (39.7835, -190.7444) (39.6723, -190.9445) (39.35, -191.3372) (39.1721, -191.5262) knots 0 0 0 1 2 2 2
  spline S188 degree 2 poles (39.1721, -191.5262) (38.8832, -191.8411) (38.1755, -192.5154) (37.9643, -192.7118) knots 0 0 0 1 2 2 2
  line L142 (37.9643, -192.7118) -> (40.2095, -192.7118)
  line L143 (40.2095, -192.7118) -> (40.2095, -193.2416)
  spline S189 degree 2 poles (43.7108, -191.7596) (43.7108, -192.1116) (43.4774, -192.7081) (43.281, -192.9082) knots 0 0 0 1 2 2 2
  spline S190 degree 2 poles (43.281, -192.9082) (43.0772, -193.1194) (42.5659, -193.338) (42.2584, -193.338) knots 0 0 0 1 2 2 2
  spline S191 degree 2 poles (42.2584, -193.338) (41.9509, -193.338) (41.4433, -193.1305) (41.2507, -192.923) knots 0 0 0 1 2 2 2
  spline S192 degree 2 poles (41.2507, -192.923) (41.0135, -192.6748) (40.7468, -191.8411) (40.7468, -191.2335) knots 0 0 0 1 2 2 2
  spline S193 degree 2 poles (40.7468, -191.2335) (40.7468, -190.637) (40.9913, -189.6774) (41.247, -189.3217) knots 0 0 0 1 2 2 2
  spline S194 degree 2 poles (41.247, -189.3217) (41.4952, -188.9734) (42.2807, -188.5844) (42.7957, -188.5844) knots 0 0 0 1 2 2 2
  spline S195 degree 2 poles (42.7957, -188.5844) (42.9476, -188.5844) (43.2143, -188.6141) (43.3144, -188.6474) knots 0 0 0 1 2 2 2
  line L144 (43.3144, -188.6474) -> (43.3144, -189.2365)
  line L145 (43.3144, -189.2365) -> (43.2884, -189.2365)
  spline S196 degree 2 poles (43.2884, -189.2365) (43.2032, -189.192) (42.892, -189.1142) (42.7141, -189.1142) knots 0 0 0 1 2 2 2
  spline S197 degree 2 poles (42.7141, -189.1142) (42.1436, -189.1142) (41.4433, -189.8849) (41.3766, -190.6407) knots 0 0 0 1 2 2 2
  spline S198 degree 2 poles (41.3766, -190.6407) (41.5952, -190.4888) (42.0547, -190.3221) (42.3288, -190.3221) knots 0 0 0 1 2 2 2
  spline S199 degree 2 poles (42.3288, -190.3221) (42.5956, -190.3221) (42.9957, -190.4295) (43.2143, -190.5925) knots 0 0 0 1 2 2 2
  spline S200 degree 2 poles (43.2143, -190.5925) (43.4663, -190.7815) (43.7108, -191.3669) (43.7108, -191.7596) knots 0 0 0 1 2 2 2
  spline S201 degree 2 poles (43.0884, -191.7856) (43.0884, -191.504) (42.9402, -191.1224) (42.7771, -190.989) knots 0 0 0 1 2 2 2
  spline S202 degree 2 poles (42.7771, -190.989) (42.6549, -190.8926) (42.3511, -190.8297) (42.1917, -190.8297) knots 0 0 0 1 2 2 2
  spline S203 degree 2 poles (42.1917, -190.8297) (41.9768, -190.8297) (41.573, -190.9593) (41.3766, -191.0816) knots 0 0 0 1 2 2 2
  spline S204 degree 2 poles (41.3766, -191.0816) (41.3729, -191.1483) (41.3655, -191.2743) (41.3655, -191.3706) knots 0 0 0 1 2 2 2
  spline S205 degree 2 poles (41.3655, -191.3706) (41.3655, -191.8448) (41.5508, -192.4265) (41.6916, -192.5784) knots 0 0 0 1 2 2 2
  spline S206 degree 2 poles (41.6916, -192.5784) (41.8212, -192.7229) (42.1028, -192.8378) (42.2621, -192.8378) knots 0 0 0 1 2 2 2
  spline S207 degree 2 poles (42.2621, -192.8378) (42.6326, -192.8378) (43.0884, -192.3117) (43.0884, -191.7856) knots 0 0 0 1 2 2 2
  point P0 (0, 0)
  constraints: 2 other
emboss "Emboss1" sketch "Sketch13" operation cut depth 2.54 direction (-1, 0, 0)